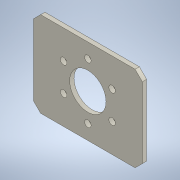
# Autodesk Inventor part: Gearbox Outer Mount
Saved by Autodesk Inventor 2022 (Build 260153000, 153)
## iProperties
Created: 2022-08-13
Part Number: Gearbox Outer Mount
Material: Steel, Galvanneal, A653 1010
Document SubType Name: Sheet Metal
Designer: Nick
Density: 7.86 g/cm^3
Sheet Metal Rule: STL A653 1010 Galvanneal .093 (13ga)
Appearance: Steel - Cast
Author: Nick
Autodesk Inventor part; units mm, degrees
ref_plane "YZ Plane" through (0, 0, 0) normal (1, 0, 0) x (0, 1, 0)
ref_plane "XZ Plane" through (0, 0, 0) normal (0, 1, 0) x (-1, 0, 0)
ref_plane "XY Plane" through (0, 0, 0) normal (0, 0, 1) x (1, 0, 0)
sketch "Sketch1" plane through (0, 0, 0) normal (0, 0, 1) x (1, 0, 0)
  line L0 (0, 0) -> (60, 0)
  line L1 (60, 0) -> (60, 47)
  line L2 (60, 47) -> (0, 47)
  line L3 (0, 47) -> (0, 0)
  circle A0 centre (30, 23.5) radius 10
  point P0 (60, 23.5)
  point P1 (30, 47)
  dimension "d0" = 60
  dimension "d1" = 47
  dimension "d2" = 20
  measures "d0" distance of L2.end L1.end
  measures "d1" distance of L1.end L0.end
  measures "d2" diameter of A0
extrude "Plate1" add sketch "Sketch1" along normal blind 2.3622
sketch "Sketch2" plane through (0, 0, 2.3622) normal (0, 0, 1) x (1, 0, 0)
  circle A0 centre (30, 23.5) radius 10 projected
  line L0 (30, 38.915) -> (30, 8.085) construction
  point P0 (0, 0)
  dimension "d4" = 30.83
  constraints: 2 end point, 2 vertical alignment, 1 coincident, 1 midpoint, 1 vertical
  measures "d4" distance of L0.end L0.start
hole "Hole1" at (30, 38.915, 2.3622) at (30, 8.085, 2.3622) direction (0, 0, -1) diameter 3.6 end through all clearance for "Flat Head Machine Screw" size "M3" standard "Ansi Metric M Profile"
pattern_circular "Circular Pattern1" count 3 over 360 about axis through (30, 23.5, 0) along (0, 0, 1) of "Hole1"
chamfer "Corner Chamfer1" distance 4 angle 45 4 edges at (0, 47, 1.1811) (0, 0, 1.1811) (60, 0, 1.1811) (60, 47, 1.1811)
equation "\"d10\" = Thickness"
equation "\"d3\" = Thickness"
equation "\"BendReliefWidth\" = Thickness"
equation "\"BendReliefDepth\" = 0.5 * Thickness"
equation "\"CornerReliefSize\" = 3 * Thickness"
equation "\"MinimumRemnant\" = 2 * Thickness"
equation "\"TransitionRadius\" = BendRadius"
equation "\"JacobiRadiusSize\" = BendRadius"
equation "\"GapSize\" = 0.5 * Thickness"
equation "\"Thickness\" = 2.3622"
equation "\"BendRadius\" = 0.79375"
body "Solid1"
